Autodesk Inventor part; units mm, degrees
(part 2 of 3)
  arc A282 (85.8723, 45.9613) -> (86.1263, 45.7073) centre (86.1263, 45.9613) ccw
  arc A283 (86.1263, 59.7027) -> (85.8723, 59.4487) centre (86.1263, 59.4487) ccw
  line L431 (85.8723, 45.7073) -> (99.8677, 59.7027) construction
  arc A284 (-19.1948, 59.4487) -> (-19.4488, 59.7027) centre (-19.4488, 59.4487) ccw
  arc A285 (-32.9362, 59.7027) -> (-33.1902, 59.4487) centre (-32.9362, 59.4487) ccw
  line L432 (-19.1948, 59.4487) -> (-19.1948, 45.9613)
  line L433 (-32.9362, 59.7027) -> (-19.4488, 59.7027)
  line L434 (-33.1902, 45.9613) -> (-33.1902, 59.4487)
  line L435 (-19.4488, 45.7073) -> (-32.9362, 45.7073)
  line L436 (-33.1902, 45.7073) -> (-19.1948, 59.7027) construction
  arc A286 (-19.4488, 45.7073) -> (-19.1948, 45.9613) centre (-19.4488, 45.9613) ccw
  arc A287 (-33.1902, 45.9613) -> (-32.9362, 45.7073) centre (-32.9362, 45.9613) ccw
  line L437 (-19.1948, 45.7073) -> (-33.1902, 59.7027) construction
  line L438 (-43.0073, 59.4487) -> (-43.0073, 45.9613)
  arc A288 (-43.2613, 45.7073) -> (-43.0073, 45.9613) centre (-43.2613, 45.9613) ccw
  arc A289 (-43.0073, 59.4487) -> (-43.2613, 59.7027) centre (-43.2613, 59.4487) ccw
  line L439 (-56.7487, 59.7027) -> (-43.2613, 59.7027)
  line L440 (-43.2613, 45.7073) -> (-56.7487, 45.7073)
  line L441 (-57.0027, 45.7073) -> (-43.0073, 59.7027) construction
  line L442 (-43.0073, 45.7073) -> (-57.0027, 59.7027) construction
  arc A290 (-56.7487, 59.7027) -> (-57.0027, 59.4487) centre (-56.7487, 59.4487) ccw
  line L443 (-57.0027, 45.9613) -> (-57.0027, 59.4487)
  arc A291 (-57.0027, 45.9613) -> (-56.7487, 45.7073) centre (-56.7487, 45.9613) ccw
  line L444 (-66.8198, 59.4487) -> (-66.8198, 45.9613)
  arc A292 (-67.0738, 45.7073) -> (-66.8198, 45.9613) centre (-67.0738, 45.9613) ccw
  arc A293 (-66.8198, 59.4487) -> (-67.0738, 59.7027) centre (-67.0738, 59.4487) ccw
  line L445 (-80.5612, 59.7027) -> (-67.0738, 59.7027)
  line L446 (-67.0738, 45.7073) -> (-80.5612, 45.7073)
  line L447 (-80.8152, 45.7073) -> (-66.8198, 59.7027) construction
  line L448 (-66.8198, 45.7073) -> (-80.8152, 59.7027) construction
  arc A294 (-80.5612, 59.7027) -> (-80.8152, 59.4487) centre (-80.5612, 59.4487) ccw
  line L449 (-80.8152, 45.9613) -> (-80.8152, 59.4487)
  arc A295 (-80.8152, 45.9613) -> (-80.5612, 45.7073) centre (-80.5612, 45.9613) ccw
  line L450 (-104.3737, 59.7027) -> (-90.8863, 59.7027)
  arc A296 (-104.3737, 59.7027) -> (-104.6277, 59.4487) centre (-104.3737, 59.4487) ccw
  arc A297 (-90.6323, 59.4487) -> (-90.8863, 59.7027) centre (-90.8863, 59.4487) ccw
  line L451 (-90.6323, 59.4487) -> (-90.6323, 45.9613)
  line L452 (-104.6277, 45.9613) -> (-104.6277, 59.4487)
  line L453 (-104.6277, 45.7073) -> (-90.6323, 59.7027) construction
  line L454 (-90.6323, 45.7073) -> (-104.6277, 59.7027) construction
  arc A298 (-90.8863, 45.7073) -> (-90.6323, 45.9613) centre (-90.8863, 45.9613) ccw
  line L455 (-90.8863, 45.7073) -> (-104.3737, 45.7073)
  arc A299 (-104.6277, 45.9613) -> (-104.3737, 45.7073) centre (-104.3737, 45.9613) ccw
  line L456 (183.1975, 52.705) -> (164.3075, 52.705) construction
  arc A300 (-121.5898, -16.7513) -> (-121.8438, -16.4973) centre (-121.8438, -16.7513) ccw
  line L457 (-121.5898, -16.7513) -> (-121.5898, -30.2387)
  arc A301 (-121.8438, -30.4927) -> (-121.5898, -30.2387) centre (-121.8438, -30.2387) ccw
  line L458 (-135.3312, -16.4973) -> (-121.8438, -16.4973)
  line L459 (-121.8438, -30.4927) -> (-135.3312, -30.4927)
  line L460 (-121.5898, -30.4927) -> (-135.5852, -16.4973) construction
  line L461 (-135.5852, -30.4927) -> (-121.5898, -16.4973) construction
  arc A302 (-135.5852, -30.2387) -> (-135.3312, -30.4927) centre (-135.3312, -30.2387) ccw
  line L462 (-135.5852, -30.2387) -> (-135.5852, -16.7513)
  arc A303 (-135.3312, -16.4973) -> (-135.5852, -16.7513) centre (-135.3312, -16.7513) ccw
  arc A304 (-121.5898, 2.2987) -> (-121.8438, 2.5527) centre (-121.8438, 2.2987) ccw
  arc A305 (-135.3312, 2.5527) -> (-135.5852, 2.2987) centre (-135.3312, 2.2987) ccw
  line L463 (-121.5898, 2.2987) -> (-121.5898, -11.1887)
  line L464 (-121.8438, -11.4427) -> (-135.3312, -11.4427)
  arc A306 (-121.8438, -11.4427) -> (-121.5898, -11.1887) centre (-121.8438, -11.1887) ccw
  line L465 (-121.5898, -11.4427) -> (-135.5852, 2.5527) construction
  line L466 (-135.5852, -11.4427) -> (-121.5898, 2.5527) construction
  line L467 (-135.5852, -11.1887) -> (-135.5852, 2.2987)
  arc A307 (-135.5852, -11.1887) -> (-135.3312, -11.4427) centre (-135.3312, -11.1887) ccw
  line L468 (-135.3312, 2.5527) -> (-121.8438, 2.5527)
  arc A308 (-121.5898, 21.3487) -> (-121.8438, 21.6027) centre (-121.8438, 21.3487) ccw
  arc A309 (-135.3312, 21.6027) -> (-135.5852, 21.3487) centre (-135.3312, 21.3487) ccw
  line L469 (-121.5898, 21.3487) -> (-121.5898, 7.8613)
  line L470 (-121.8438, 7.6073) -> (-135.3312, 7.6073)
  arc A310 (-121.8438, 7.6073) -> (-121.5898, 7.8613) centre (-121.8438, 7.8613) ccw
  line L471 (-121.5898, 7.6073) -> (-135.5852, 21.6027) construction
  line L472 (-135.5852, 7.6073) -> (-121.5898, 21.6027) construction
  line L473 (-135.5852, 7.8613) -> (-135.5852, 21.3487)
  arc A311 (-135.5852, 7.8613) -> (-135.3312, 7.6073) centre (-135.3312, 7.8613) ccw
  line L474 (-135.3312, 21.6027) -> (-121.8438, 21.6027)
  arc A312 (-121.5898, 40.3987) -> (-121.8438, 40.6527) centre (-121.8438, 40.3987) ccw
  arc A313 (-135.3312, 40.6527) -> (-135.5852, 40.3987) centre (-135.3312, 40.3987) ccw
  line L475 (-121.5898, 40.3987) -> (-121.5898, 26.9113)
  line L476 (-121.8438, 26.6573) -> (-135.3312, 26.6573)
  arc A314 (-121.8438, 26.6573) -> (-121.5898, 26.9113) centre (-121.8438, 26.9113) ccw
  line L477 (-121.5898, 26.6573) -> (-135.5852, 40.6527) construction
  line L478 (-135.5852, 26.6573) -> (-121.5898, 40.6527) construction
  line L479 (-135.5852, 26.9113) -> (-135.5852, 40.3987)
  arc A315 (-135.5852, 26.9113) -> (-135.3312, 26.6573) centre (-135.3312, 26.9113) ccw
  line L480 (-135.3312, 40.6527) -> (-121.8438, 40.6527)
  arc A316 (-121.5898, 59.4487) -> (-121.8438, 59.7027) centre (-121.8438, 59.4487) ccw
  arc A317 (-135.3312, 59.7027) -> (-135.5852, 59.4487) centre (-135.3312, 59.4487) ccw
  line L481 (-121.5898, 59.4487) -> (-121.5898, 45.9613)
  line L482 (-121.8438, 45.7073) -> (-135.3312, 45.7073)
  arc A318 (-121.8438, 45.7073) -> (-121.5898, 45.9613) centre (-121.8438, 45.9613) ccw
  line L483 (-121.5898, 45.7073) -> (-135.5852, 59.7027) construction
  line L484 (-135.5852, 45.7073) -> (-121.5898, 59.7027) construction
  line L485 (-135.5852, 45.9613) -> (-135.5852, 59.4487)
  arc A319 (-135.5852, 45.9613) -> (-135.3312, 45.7073) centre (-135.3312, 45.9613) ccw
  line L486 (-135.3312, 59.7027) -> (-121.8438, 59.7027)
  arc A320 (-140.6398, -16.7513) -> (-140.8938, -16.4973) centre (-140.8938, -16.7513) ccw
  arc A321 (-154.3812, -16.4973) -> (-154.6352, -16.7513) centre (-154.3812, -16.7513) ccw
  line L487 (-140.6398, -16.7513) -> (-140.6398, -30.2387)
  line L488 (-140.8938, -30.4927) -> (-154.3812, -30.4927)
  arc A322 (-140.8938, -30.4927) -> (-140.6398, -30.2387) centre (-140.8938, -30.2387) ccw
  line L489 (-140.6398, -30.4927) -> (-154.6352, -16.4973) construction
  line L490 (-154.6352, -30.4927) -> (-140.6398, -16.4973) construction
  line L491 (-154.6352, -30.2387) -> (-154.6352, -16.7513)
  arc A323 (-154.6352, -30.2387) -> (-154.3812, -30.4927) centre (-154.3812, -30.2387) ccw
  line L492 (-154.3812, -16.4973) -> (-140.8938, -16.4973)
  arc A324 (-140.6398, 2.2987) -> (-140.8938, 2.5527) centre (-140.8938, 2.2987) ccw
  arc A325 (-154.3812, 2.5527) -> (-154.6352, 2.2987) centre (-154.3812, 2.2987) ccw
  line L493 (-140.6398, 2.2987) -> (-140.6398, -11.1887)
  line L494 (-140.8938, -11.4427) -> (-154.3812, -11.4427)
  arc A326 (-140.8938, -11.4427) -> (-140.6398, -11.1887) centre (-140.8938, -11.1887) ccw
  line L495 (-140.6398, -11.4427) -> (-154.6352, 2.5527) construction
  line L496 (-154.6352, -11.4427) -> (-140.6398, 2.5527) construction
  line L497 (-154.6352, -11.1887) -> (-154.6352, 2.2987)
  arc A327 (-154.6352, -11.1887) -> (-154.3812, -11.4427) centre (-154.3812, -11.1887) ccw
  line L498 (-154.3812, 2.5527) -> (-140.8938, 2.5527)
  arc A328 (-140.6398, 21.3487) -> (-140.8938, 21.6027) centre (-140.8938, 21.3487) ccw
  arc A329 (-154.3812, 21.6027) -> (-154.6352, 21.3487) centre (-154.3812, 21.3487) ccw
  line L499 (-140.6398, 21.3487) -> (-140.6398, 7.8613)
  line L500 (-140.8938, 7.6073) -> (-154.3812, 7.6073)
  arc A330 (-140.8938, 7.6073) -> (-140.6398, 7.8613) centre (-140.8938, 7.8613) ccw
  line L501 (-140.6398, 7.6073) -> (-154.6352, 21.6027) construction
  line L502 (-154.6352, 7.6073) -> (-140.6398, 21.6027) construction
  line L503 (-154.6352, 7.8613) -> (-154.6352, 21.3487)
  arc A331 (-154.6352, 7.8613) -> (-154.3812, 7.6073) centre (-154.3812, 7.8613) ccw
  line L504 (-154.3812, 21.6027) -> (-140.8938, 21.6027)
  arc A332 (-140.6398, 40.3987) -> (-140.8938, 40.6527) centre (-140.8938, 40.3987) ccw
  arc A333 (-154.3812, 40.6527) -> (-154.6352, 40.3987) centre (-154.3812, 40.3987) ccw
  line L505 (-140.6398, 40.3987) -> (-140.6398, 26.9113)
  line L506 (-140.8938, 26.6573) -> (-154.3812, 26.6573)
  arc A334 (-140.8938, 26.6573) -> (-140.6398, 26.9113) centre (-140.8938, 26.9113) ccw
  line L507 (-140.6398, 26.6573) -> (-154.6352, 40.6527) construction
  line L508 (-154.6352, 26.6573) -> (-140.6398, 40.6527) construction
  line L509 (-154.6352, 26.9113) -> (-154.6352, 40.3987)
  arc A335 (-154.6352, 26.9113) -> (-154.3812, 26.6573) centre (-154.3812, 26.9113) ccw
  line L510 (-154.3812, 40.6527) -> (-140.8938, 40.6527)
  arc A336 (-140.6398, 59.4487) -> (-140.8938, 59.7027) centre (-140.8938, 59.4487) ccw
  arc A337 (-154.3812, 59.7027) -> (-154.6352, 59.4487) centre (-154.3812, 59.4487) ccw
  line L511 (-140.6398, 59.4487) -> (-140.6398, 45.9613)
  line L512 (-140.8938, 45.7073) -> (-154.3812, 45.7073)
  arc A338 (-140.8938, 45.7073) -> (-140.6398, 45.9613) centre (-140.8938, 45.9613) ccw
  line L513 (-140.6398, 45.7073) -> (-154.6352, 59.7027) construction
  line L514 (-154.6352, 45.7073) -> (-140.6398, 59.7027) construction
  line L515 (-154.6352, 45.9613) -> (-154.6352, 59.4487)
  arc A339 (-154.6352, 45.9613) -> (-154.3812, 45.7073) centre (-154.3812, 45.9613) ccw
  line L516 (-154.3812, 59.7027) -> (-140.8938, 59.7027)
  arc A340 (-159.6898, -16.7513) -> (-159.9438, -16.4973) centre (-159.9438, -16.7513) ccw
  arc A341 (-173.4312, -16.4973) -> (-173.6852, -16.7513) centre (-173.4312, -16.7513) ccw
  line L517 (-159.6898, -16.7513) -> (-159.6898, -30.2387)
  line L518 (-159.9438, -30.4927) -> (-173.4312, -30.4927)
  arc A342 (-159.9438, -30.4927) -> (-159.6898, -30.2387) centre (-159.9438, -30.2387) ccw
  line L519 (-159.6898, -30.4927) -> (-173.6852, -16.4973) construction
  line L520 (-173.6852, -30.4927) -> (-159.6898, -16.4973) construction
  line L521 (-173.6852, -30.2387) -> (-173.6852, -16.7513)
  arc A343 (-173.6852, -30.2387) -> (-173.4312, -30.4927) centre (-173.4312, -30.2387) ccw
  line L522 (-173.4312, -16.4973) -> (-159.9438, -16.4973)
  arc A344 (-159.6898, 2.2987) -> (-159.9438, 2.5527) centre (-159.9438, 2.2987) ccw
  arc A345 (-173.4312, 2.5527) -> (-173.6852, 2.2987) centre (-173.4312, 2.2987) ccw
  line L523 (-159.6898, 2.2987) -> (-159.6898, -11.1887)
  line L524 (-159.9438, -11.4427) -> (-173.4312, -11.4427)
  arc A346 (-159.9438, -11.4427) -> (-159.6898, -11.1887) centre (-159.9438, -11.1887) ccw
  line L525 (-159.6898, -11.4427) -> (-173.6852, 2.5527) construction
  line L526 (-173.6852, -11.4427) -> (-159.6898, 2.5527) construction
  line L527 (-173.6852, -11.1887) -> (-173.6852, 2.2987)
  arc A347 (-173.6852, -11.1887) -> (-173.4312, -11.4427) centre (-173.4312, -11.1887) ccw
  line L528 (-173.4312, 2.5527) -> (-159.9438, 2.5527)
  arc A348 (-159.6898, 21.3487) -> (-159.9438, 21.6027) centre (-159.9438, 21.3487) ccw
  arc A349 (-173.4312, 21.6027) -> (-173.6852, 21.3487) centre (-173.4312, 21.3487) ccw
  line L529 (-159.6898, 21.3487) -> (-159.6898, 7.8613)
  line L530 (-159.9438, 7.6073) -> (-173.4312, 7.6073)
  arc A350 (-159.9438, 7.6073) -> (-159.6898, 7.8613) centre (-159.9438, 7.8613) ccw
  line L531 (-159.6898, 7.6073) -> (-173.6852, 21.6027) construction
  line L532 (-173.6852, 7.6073) -> (-159.6898, 21.6027) construction
  line L533 (-173.6852, 7.8613) -> (-173.6852, 21.3487)
  arc A351 (-173.6852, 7.8613) -> (-173.4312, 7.6073) centre (-173.4312, 7.8613) ccw
  line L534 (-173.4312, 21.6027) -> (-159.9438, 21.6027)
  arc A352 (-159.6898, 40.3987) -> (-159.9438, 40.6527) centre (-159.9438, 40.3987) ccw
  arc A353 (-173.4312, 40.6527) -> (-173.6852, 40.3987) centre (-173.4312, 40.3987) ccw
  line L535 (-159.6898, 40.3987) -> (-159.6898, 26.9113)
  line L536 (-159.9438, 26.6573) -> (-173.4312, 26.6573)
  arc A354 (-159.9438, 26.6573) -> (-159.6898, 26.9113) centre (-159.9438, 26.9113) ccw
  line L537 (-159.6898, 26.6573) -> (-173.6852, 40.6527) construction
  line L538 (-173.6852, 26.6573) -> (-159.6898, 40.6527) construction
  line L539 (-173.6852, 26.9113) -> (-173.6852, 40.3987)
  arc A355 (-173.6852, 26.9113) -> (-173.4312, 26.6573) centre (-173.4312, 26.9113) ccw
  line L540 (-173.4312, 40.6527) -> (-159.9438, 40.6527)
  arc A356 (-159.6898, 59.4487) -> (-159.9438, 59.7027) centre (-159.9438, 59.4487) ccw
  arc A357 (-173.4312, 59.7027) -> (-173.6852, 59.4487) centre (-173.4312, 59.4487) ccw
  line L541 (-159.6898, 59.4487) -> (-159.6898, 45.9613)
  line L542 (-159.9438, 45.7073) -> (-173.4312, 45.7073)
  arc A358 (-159.9438, 45.7073) -> (-159.6898, 45.9613) centre (-159.9438, 45.9613) ccw
  line L543 (-159.6898, 45.7073) -> (-173.6852, 59.7027) construction
  line L544 (-173.6852, 45.7073) -> (-159.6898, 59.7027) construction
  line L545 (-173.6852, 45.9613) -> (-173.6852, 59.4487)
  arc A359 (-173.6852, 45.9613) -> (-173.4312, 45.7073) centre (-173.4312, 45.9613) ccw
  line L546 (-173.4312, 59.7027) -> (-159.9438, 59.7027)
  line L547 (-100.0125, -23.495) -> (-183.1975, -23.495) construction
  line L548 (24.5491, 47.3329) -> (18.0571, 47.3329)
  line L549 (17.8031, 47.5869) -> (17.8031, 58.5089)
  line L550 (18.0571, 58.7629) -> (24.5491, 58.7629)
  line L551 (24.8031, 58.5089) -> (24.8031, 47.5869)
  line L552 (21.3031, 47.3329) -> (21.3031, 52.705) construction
  line L553 (33.3375, 59.7027) -> (33.3375, 45.7073) construction
  line L554 (42.1259, 47.3329) -> (48.6179, 47.3329)
  line L555 (48.8719, 47.5869) -> (48.8719, 58.5089)
  line L556 (48.6179, 58.7629) -> (42.1259, 58.7629)
  line L557 (41.8719, 58.5089) -> (41.8719, 47.5869)
  line L558 (45.3719, 47.3329) -> (45.3719, 52.705) construction
  line L559 (150.1648, 26.9113) -> (150.1648, 40.3987)
  line L560 (150.4188, 40.6527) -> (163.9062, 40.6527)
  line L561 (164.1602, 26.6573) -> (150.1648, 40.6527) construction
  line L562 (164.1602, 40.6527) -> (150.1648, 26.6573) construction
  line L563 (148.3741, 28.2829) -> (141.8821, 28.2829)
  line L564 (141.6281, 28.5369) -> (141.6281, 39.4589)
  line L565 (141.8821, 39.7129) -> (148.3741, 39.7129)
  line L566 (148.6281, 39.4589) -> (148.6281, 28.5369)
  line L567 (145.1281, 28.2829) -> (145.1281, 33.655) construction
  line L568 (157.1625, 33.655) -> (145.1281, 33.655) construction
  line L569 (157.1625, 26.6573) -> (157.1625, 40.6527) construction
  line L570 (172.4429, 39.7129) -> (165.9509, 39.7129)
  line L571 (172.6969, 28.5369) -> (172.6969, 39.4589)
  line L572 (169.1969, 28.2829) -> (169.1969, 33.655) construction
  line L573 (165.9509, 28.2829) -> (172.4429, 28.2829)
  line L574 (165.6969, 39.4589) -> (165.6969, 28.5369)
  line L575 (11.1835, 47.3329) -> (4.6915, 47.3329)
  line L576 (4.4375, 47.5869) -> (4.4375, 58.5089)
  line L577 (4.6915, 58.7629) -> (11.1835, 58.7629)
  line L578 (11.4375, 58.5089) -> (11.4375, 47.5869)
  line L579 (7.9375, 47.3329) -> (7.9375, 58.7629) construction
  line L580 (55.4915, 47.3329) -> (61.9835, 47.3329)
  line L581 (62.2375, 47.5869) -> (62.2375, 58.5089)
  line L582 (61.9835, 58.7629) -> (55.4915, 58.7629)
  line L583 (55.2375, 58.5089) -> (55.2375, 47.5869)
  line L584 (58.7375, 47.3329) -> (58.7375, 58.7629) construction
  line L585 (150.4188, 26.6573) -> (163.9062, 26.6573)
  line L586 (164.1602, 40.3987) -> (164.1602, 26.9113)
  arc A360 (163.9062, 26.6573) -> (164.1602, 26.9113) centre (163.9062, 26.9113) ccw
  arc A361 (164.1602, 40.3987) -> (163.9062, 40.6527) centre (163.9062, 40.3987) ccw
  arc A362 (150.4188, 40.6527) -> (150.1648, 40.3987) centre (150.4188, 40.3987) ccw
  arc A363 (150.1648, 26.9113) -> (150.4188, 26.6573) centre (150.4188, 26.9113) ccw
  arc A364 (172.4429, 28.2829) -> (172.6969, 28.5369) centre (172.4429, 28.5369) ccw
  arc A365 (172.6969, 39.4589) -> (172.4429, 39.7129) centre (172.4429, 39.4589) ccw
  arc A366 (165.9509, 39.7129) -> (165.6969, 39.4589) centre (165.9509, 39.4589) ccw
  arc A367 (165.6969, 28.5369) -> (165.9509, 28.2829) centre (165.9509, 28.5369) ccw
  arc A368 (148.3741, 28.2829) -> (148.6281, 28.5369) centre (148.3741, 28.5369) ccw
  arc A369 (148.6281, 39.4589) -> (148.3741, 39.7129) centre (148.3741, 39.4589) ccw
  arc A370 (141.8821, 39.7129) -> (141.6281, 39.4589) centre (141.8821, 39.4589) ccw
  arc A371 (141.6281, 28.5369) -> (141.8821, 28.2829) centre (141.8821, 28.5369) ccw
  line L587 (40.0812, 45.7073) -> (26.5938, 45.7073)
  line L588 (26.3398, 45.9613) -> (26.3398, 59.4487)
  line L589 (26.5938, 59.7027) -> (40.0812, 59.7027)
  line L590 (40.3352, 59.4487) -> (40.3352, 45.9613)
  line L591 (40.3352, 45.7073) -> (26.3398, 59.7027) construction
  line L592 (40.3352, 59.7027) -> (26.3398, 45.7073) construction
  arc A372 (40.0812, 45.7073) -> (40.3352, 45.9613) centre (40.0812, 45.9613) ccw
  arc A373 (40.3352, 59.4487) -> (40.0812, 59.7027) centre (40.0812, 59.4487) ccw
  arc A374 (26.5938, 59.7027) -> (26.3398, 59.4487) centre (26.5938, 59.4487) ccw
  arc A375 (26.3398, 45.9613) -> (26.5938, 45.7073) centre (26.5938, 45.9613) ccw
  arc A376 (48.6179, 47.3329) -> (48.8719, 47.5869) centre (48.6179, 47.5869) ccw
  arc A377 (48.8719, 58.5089) -> (48.6179, 58.7629) centre (48.6179, 58.5089) ccw
  arc A378 (42.1259, 58.7629) -> (41.8719, 58.5089) centre (42.1259, 58.5089) ccw
  arc A379 (41.8719, 47.5869) -> (42.1259, 47.3329) centre (42.1259, 47.5869) ccw
  arc A380 (24.5491, 47.3329) -> (24.8031, 47.5869) centre (24.5491, 47.5869) ccw
  arc A381 (17.8031, 47.5869) -> (18.0571, 47.3329) centre (18.0571, 47.5869) ccw
  arc A382 (18.0571, 58.7629) -> (17.8031, 58.5089) centre (18.0571, 58.5089) ccw
  arc A383 (24.8031, 58.5089) -> (24.5491, 58.7629) centre (24.5491, 58.5089) ccw
  arc A384 (11.1835, 47.3329) -> (11.4375, 47.5869) centre (11.1835, 47.5869) ccw
  arc A385 (4.4375, 47.5869) -> (4.6915, 47.3329) centre (4.6915, 47.5869) ccw
  arc A386 (4.6915, 58.7629) -> (4.4375, 58.5089) centre (4.6915, 58.5089) ccw
  arc A387 (11.4375, 58.5089) -> (11.1835, 58.7629) centre (11.1835, 58.5089) ccw
  arc A388 (55.2375, 47.5869) -> (55.4915, 47.3329) centre (55.4915, 47.5869) ccw
  arc A389 (61.9835, 47.3329) -> (62.2375, 47.5869) centre (61.9835, 47.5869) ccw
  arc A390 (62.2375, 58.5089) -> (61.9835, 58.7629) centre (61.9835, 58.5089) ccw
  arc A391 (55.4915, 58.7629) -> (55.2375, 58.5089) centre (55.4915, 58.5089) ccw
  line L593 (21.3031, 52.705) -> (33.3375, 52.705) construction
  line L594 (-83.7438, 26.6573) -> (-97.2312, 26.6573)
  line L595 (-97.4852, 26.9113) -> (-97.4852, 40.3987)
  line L596 (-97.2312, 40.6527) -> (-83.7438, 40.6527)
  line L597 (-83.4898, 40.3987) -> (-83.4898, 26.9113)
  line L598 (-83.4898, 26.6573) -> (-97.4852, 40.6527) construction
  line L599 (-97.4852, 26.6573) -> (-83.4898, 40.6527) construction
  arc A392 (-83.7438, 26.6573) -> (-83.4898, 26.9113) centre (-83.7438, 26.9113) ccw
  arc A393 (-97.4852, 26.9113) -> (-97.2312, 26.6573) centre (-97.2312, 26.9113) ccw
  arc A394 (-97.2312, 40.6527) -> (-97.4852, 40.3987) centre (-97.2312, 40.3987) ccw
  arc A395 (-83.4898, 40.3987) -> (-83.7438, 40.6527) centre (-83.7438, 40.3987) ccw
  line L600 (-90.4875, 26.6573) -> (-90.4875, 40.6527) construction
  line L601 (-99.2759, 28.2829) -> (-105.7679, 28.2829)
  line L602 (-106.0219, 28.5369) -> (-106.0219, 39.4589)
  line L603 (-105.7679, 39.7129) -> (-99.2759, 39.7129)
  line L604 (-99.0219, 39.4589) -> (-99.0219, 28.5369)
  arc A396 (-99.2759, 28.2829) -> (-99.0219, 28.5369) centre (-99.2759, 28.5369) ccw
  arc A397 (-106.0219, 28.5369) -> (-105.7679, 28.2829) centre (-105.7679, 28.5369) ccw
  arc A398 (-105.7679, 39.7129) -> (-106.0219, 39.4589) centre (-105.7679, 39.4589) ccw
  arc A399 (-99.0219, 39.4589) -> (-99.2759, 39.7129) centre (-99.2759, 39.4589) ccw
  line L605 (-81.6991, 28.2829) -> (-75.2071, 28.2829)
  line L606 (-74.9531, 28.5369) -> (-74.9531, 39.4589)
  line L607 (-75.2071, 39.7129) -> (-81.6991, 39.7129)
  line L608 (-81.9531, 39.4589) -> (-81.9531, 28.5369)
  arc A400 (-81.9531, 28.5369) -> (-81.6991, 28.2829) centre (-81.6991, 28.5369) ccw
  arc A401 (-75.2071, 28.2829) -> (-74.9531, 28.5369) centre (-75.2071, 28.5369) ccw
  arc A402 (-74.9531, 39.4589) -> (-75.2071, 39.7129) centre (-75.2071, 39.4589) ccw
  arc A403 (-81.6991, 39.7129) -> (-81.9531, 39.4589) centre (-81.6991, 39.4589) ccw
  line L609 (-78.4531, 28.2829) -> (-78.4531, 33.655) construction
  line L610 (-102.5219, 28.2829) -> (-102.5219, 33.655) construction
  line L611 (-102.5219, 33.655) -> (-78.4531, 33.655) construction
  arc A404 (-90.6323, 11.8237) -> (-90.8863, 12.0777) centre (-90.8863, 11.8237) ccw
  line L612 (-90.6323, 11.8237) -> (-90.6323, -1.6637)
  arc A405 (-90.8863, -1.9177) -> (-90.6323, -1.6637) centre (-90.8863, -1.6637) ccw
  line L613 (-104.3737, 12.0777) -> (-90.8863, 12.0777)
  line L614 (-90.8863, -1.9177) -> (-104.3737, -1.9177)
  line L615 (-90.6323, -1.9177) -> (-104.6277, 12.0777) construction
  line L616 (-104.6277, -1.9177) -> (-90.6323, 12.0777) construction
  arc A406 (-104.6277, -1.6637) -> (-104.3737, -1.9177) centre (-104.3737, -1.6637) ccw
  line L617 (-104.6277, -1.6637) -> (-104.6277, 11.8237)
  arc A407 (-104.3737, 12.0777) -> (-104.6277, 11.8237) centre (-104.3737, 11.8237) ccw
  line L618 (-92.5119, -10.2616) -> (-103.4339, -10.2616)
  line L619 (-103.6879, -10.0076) -> (-103.6879, -3.7084)
  line L620 (-103.4339, -3.4544) -> (-92.5119, -3.4544)
  line L621 (-92.2579, -3.7084) -> (-92.2579, -10.0076)
  line L622 (-92.2579, -6.858) -> (-97.63, -6.858) construction
  line L623 (-90.6323, 5.08) -> (-104.6277, 5.08) construction
  line L624 (-97.63, -6.858) -> (-97.63, 5.08) construction
  arc A408 (-92.5119, -10.2616) -> (-92.2579, -10.0076) centre (-92.5119, -10.0076) ccw
  arc A409 (-103.6879, -10.0076) -> (-103.4339, -10.2616) centre (-103.4339, -10.0076) ccw
  arc A410 (-103.4339, -3.4544) -> (-103.6879, -3.7084) centre (-103.4339, -3.7084) ccw
  arc A411 (-92.2579, -3.7084) -> (-92.5119, -3.4544) centre (-92.5119, -3.7084) ccw
  line L625 (-92.5119, 20.4216) -> (-103.4339, 20.4216)
  line L626 (-103.6879, 20.1676) -> (-103.6879, 13.8684)
  line L627 (-103.4339, 13.6144) -> (-92.5119, 13.6144)
  line L628 (-92.2579, 13.8684) -> (-92.2579, 20.1676)
  line L629 (-92.2579, 17.018) -> (-97.63, 17.018) construction
  arc A412 (-92.2579, 20.1676) -> (-92.5119, 20.4216) centre (-92.5119, 20.1676) ccw
  arc A413 (-103.4339, 20.4216) -> (-103.6879, 20.1676) centre (-103.4339, 20.1676) ccw
  arc A414 (-103.6879, 13.8684) -> (-103.4339, 13.6144) centre (-103.4339, 13.8684) ccw
  arc A415 (-92.5119, 13.6144) -> (-92.2579, 13.8684) centre (-92.5119, 13.8684) ccw
  point P0 (0, 0)
  point P1 (0, 0)
  point P2 (166.6875, -23.495)
  point P3 (69.9269, -109.0243)
  point P4 (166.6875, -52.07)
  point P5 (166.6875, -52.07)
  point P6 (147.6375, -23.495)
  point P7 (128.5875, -23.495)
  point P8 (109.5375, -23.495)
  point P9 (90.4875, -23.495)
  point P10 (71.4375, -23.495)
  point P11 (52.3875, -23.495)
  point P12 (33.3375, -23.495)
  point P13 (14.2875, -23.495)
  point P14 (-4.7625, -23.495)
  point P15 (-23.8125, -23.495)
  point P16 (-42.8625, -23.495)
  point P17 (-61.9125, -23.495)
  point P18 (-80.9625, -23.495)
  point P19 (166.6875, -23.495)
  point P20 (138.1125, -4.445)
  point P21 (119.0625, -4.445)
  point P22 (100.0125, -4.445)
  point P23 (80.9625, -4.445)
  point P24 (61.9125, -4.445)
  point P25 (42.8625, -4.445)
  point P26 (23.8125, -4.445)
  point P27 (4.7625, -4.445)
  point P28 (-14.2875, -4.445)
  point P29 (-33.3375, -4.445)
  point P30 (-52.3875, -4.445)
  point P31 (-71.4375, -4.445)
  point P32 (133.35, 14.605)
  point P33 (114.3, 14.605)
  point P34 (95.25, 14.605)
  point P35 (76.2, 14.605)
  point P36 (57.15, 14.605)
  point P37 (38.1, 14.605)
  point P38 (19.05, 14.605)
  point P39 (0, 14.605)
  point P40 (-19.05, 14.605)
  point P41 (-38.1, 14.605)
  point P42 (-57.15, 14.605)
  point P43 (-76.2, 14.605)
  point P44 (159.5425, 14.605)
  point P45 (159.5425, 14.605)
  point P46 (161.925, -4.445)
  point P47 (161.925, -4.445)
  point P48 (109.5375, 33.655)
  point P49 (90.4875, 33.655)
  point P50 (71.4375, 33.655)
  point P51 (52.3875, 33.655)
  point P52 (33.3375, 33.655)
  point P53 (14.2875, 33.655)
  point P54 (-4.7625, 33.655)
  point P55 (-23.8125, 33.655)
  point P56 (-42.8625, 33.655)
  point P57 (-61.9125, 33.655)
  point P58 (140.495, 52.705)
  point P59 (116.6825, 52.705)
  point P60 (92.87, 52.705)
  point P61 (-26.1925, 52.705)
  point P62 (-50.005, 52.705)
  point P63 (-73.8175, 52.705)
  point P64 (-97.63, 52.705)
  point P65 (-128.5875, -23.495)
  point P66 (-128.5875, -4.445)
  point P67 (-128.5875, 14.605)
  point P68 (-128.5875, 33.655)
  point P69 (-128.5875, 52.705)
  point P70 (-147.6375, -23.495)
  point P71 (-147.6375, -4.445)
  point P72 (-147.6375, 14.605)
  point P73 (-147.6375, 33.655)
  point P74 (-147.6375, 52.705)
  point P75 (-166.6875, -23.495)
  point P76 (-166.6875, -4.445)
  point P77 (-166.6875, 14.605)
  point P78 (-166.6875, 33.655)
  point P79 (-166.6875, 52.705)
  point P80 (-128.5875, -23.495)
  point P81 (24.8031, 47.3329)
  point P82 (17.8031, 58.7629)
  point P83 (17.8031, 47.3329)
  point P84 (24.8031, 58.7629)
  point P85 (41.8719, 47.3329)
  point P86 (48.8719, 58.7629)
  point P87 (48.8719, 47.3329)
  point P88 (41.8719, 58.7629)
  point P89 (148.6281, 28.2829)
  point P90 (141.6281, 39.7129)
  point P91 (141.6281, 28.2829)
  point P92 (148.6281, 39.7129)
  point P93 (172.6969, 39.7129)
  point P94 (165.6969, 39.7129)
  point P95 (172.6969, 28.2829)
  point P96 (165.6969, 28.2829)
  point P97 (157.1625, 33.655)
  point P98 (-97.63, 5.08)
  point P99 (11.4375, 47.3329)
  point P100 (4.4375, 58.7629)
  point P101 (4.4375, 47.3329)
  point P102 (11.4375, 58.7629)
  point P103 (55.2375, 47.3329)
  point P104 (62.2375, 58.7629)
  point P105 (62.2375, 47.3329)
  point P106 (55.2375, 58.7629)
  point P107 (-90.4875, 33.655)
  point P108 (26.3398, 59.7027)
  point P109 (-83.4898, 40.6527)
  point P110 (-90.4875, 33.655)
  point P111 (-106.0219, 39.7129)
  point P112 (-106.0219, 28.2829)
  point P113 (-99.0219, 39.7129)
  point P114 (-74.9531, 39.7129)
  point P115 (-74.9531, 28.2829)
  point P116 (-81.9531, 39.7129)
  point P117 (-90.4875, 33.655)
  point P118 (-90.4875, 33.655)
  point P119 (-97.63, 5.08)
  point P120 (-103.6879, -3.4544)
  point P121 (-103.6879, -10.2616)
  point P122 (-92.2579, -3.4544)
  point P123 (-103.6879, 13.6144)
  point P124 (-103.6879, 20.4216)
  point P125 (-92.2579, 13.6144)
  point P126 (-97.63, 5.08)
  dimension "d0" = 366.395
  dimension "d1" = 137.16
  dimension "d2" = 3
  dimension "d3" = 13.9954
  dimension "d4" = 13.9954
  dimension "d5" = 0.254
  dimension "d8" = 19.05
  dimension "d15" = 85.725
  dimension "d20" = 54.61
  dimension "d21" = 16.51
  dimension "d26" = 13.9954
  dimension "d27" = 13.9954
  dimension "d28" = 0.254
  dimension "d29" = 13.9954
  dimension "d30" = 13.9954
  dimension "d31" = 0.254
  dimension "d32" = 13.9954
  dimension "d33" = 13.9954
  dimension "d34" = 0.254
  dimension "d35" = 13.9954
  dimension "d36" = 13.9954
  dimension "d37" = 0.254
  dimension "d39" = 28.575
  dimension "d42" = 19.05
  dimension "d47" = 16.51
  dimension "d48" = 13.9954
  dimension "d49" = 13.9954
  dimension "d50" = 0.254
  dimension "d53" = 19.05
  dimension "d58" = 45.085
  dimension "d59" = 19.05
  dimension "d60" = 13.9954
  dimension "d61" = 13.9954
  dimension "d62" = 0.254
  dimension "d65" = 19.05
  dimension "d70" = 49.8475
  dimension "d71" = 23.655
  dimension "d72" = 19.05
  dimension "d73" = 13.9954
  dimension "d74" = 13.9954
  dimension "d75" = 0.254
  dimension "d76" = 21.2725
  dimension "d77" = 13.9954
  dimension "d78" = 13.9954
  dimension "d79" = 0.254
  dimension "d82" = 19.05
  dimension "d87" = 54.61
  dimension "d92" = 19.05
  dimension "d93" = 26.035
  dimension "d94" = 13.9954
  dimension "d95" = 13.9954
  dimension "d96" = 0.254
  dimension "d99" = 23.8125
  dimension "d106" = 190.5
  dimension "d111" = 18.89
  dimension "d112" = 19.05
  dimension "d113" = 13.9954
  dimension "d114" = 13.9954
  dimension "d115" = 0.254
  dimension "d118" = 19.05
  dimension "d121" = 19.05
  dimension "d124" = 28.575
  dimension "d145" = 7
  dimension "d146" = 11.43
  constraints: 1258 end point, 835 point on line, 832 point on circle, 416 centre point, 190 tangent, 74 equal radius, 52 symmetric about line, 47 midpoint, 40 parallel, 39 horizontal, 24 perpendicular, 16 collinear, 7 coincident, 7 vertical, 2105 other
  measures "d0" distance of L5.end L4.start
  measures "d1" distance of L4.end L5.end
  measures "d2" radius of A0
  measures "d3" distance of L10.end L11.end
  measures "d4" distance of L11.start L10.end
  measures "d5" radius of A4
  measures "d8" distance of L10.start L15.start
  measures "d15" distance of L10.end L33.end
  measures "d21" distance between parallel lines of L0 L79
  measures "d26" distance of L84.end L85.end
  measures "d27" distance of L85.start L84.end
  measures "d28" radius of A52
  measures "d29" distance of L90.end L91.end
  measures "d30" distance of L91.start L90.end
  measures "d31" radius of A56
  measures "d32" distance of L96.end L97.end
  measures "d33" distance of L97.start L96.end
  measures "d34" radius of A60
  measures "d35" distance of L101.end L102.end
  measures "d36" distance of L102.start L101.end
  measures "d37" radius of A65
  measures "d39" distance of point (166.688, -52.07) point (166.688, -23.495)
  measures "d42" distance of L84.start L108.start
  measures "d48" distance of L192.end L193.end
  measures "d49" distance of L193.start L192.end
  measures "d50" radius of A127
  measures "d53" distance of L192.end L199.end
  measures "d58" distance of L261.end L261.start
  measures "d59" distance from line of L261 point (166.688, -23.495)
  measures "d60" distance of L265.end L266.end
  measures "d61" distance of L266.start L265.end
  measures "d62" radius of A175
  measures "d65" distance of A174.centre A176.centre
  measures "d70" distance of L334.end L334.start
  measures "d72" distance between parallel lines of L334 L261
  measures "d73" distance of L338.end L339.end
  measures "d74" distance of L339.start L338.end
  measures "d75" radius of A223
  measures "d77" distance of L344.end L345.end
  measures "d78" distance of L345.start L344.end
  measures "d79" radius of A227
  measures "d82" distance of L99.end L349.end
  measures "d87" distance of L407.end L407.start
  measures "d92" distance between parallel lines of L334 L407
  measures "d94" distance of L411.end L412.end
  measures "d95" distance of L412.start L411.end
  measures "d96" radius of A269
  measures "d99" distance of L408.start L414.start
  measures "d106" distance of L408.end L432.end
  measures "d111" distance of L456.end L456.start
  measures "d112" distance between parallel lines of L407 L456
  measures "d113" distance of L460.end L461.end
  measures "d114" distance of L461.start L460.end
  measures "d115" radius of A301
  measures "d118" distance of L458.end L468.end
  measures "d121" distance of L458.end L492.end
  measures "d124" distance of point (-128.587, -23.495) L547.start
  measures "d145" distance of point (17.803, 58.763) point (24.803, 58.763)
  measures "d146" distance of point (17.803, 47.333) point (17.803, 58.763)
extrude "押し出し1" add sketch "スケッチ1" along normal blind 1.524 contours L0 A3 L1 A2 L2 A1 L3 A0 | L469 A310 L470 A311 L473 A309 L474 A308 | L475 A314 L476 A315 L479 A313 L480 A312 | L499 A330 L500 A331 L503 A329 L504 A328 | L529 A350 L530 A351 L533 A349 L534 A348 | L535 A354 L536 A355 L539 A353 L540 A352
fillet "フィレット1" radius 0.1 16 edges at (182.3188, 1.524, 67.7013) (183.1975, 1.524, 0) (182.3188, 1.524, -67.7013) (0, 1.524, -68.58) (-182.3188, 1.524, -67.7013) (-183.1975, 1.524, 0) (-182.3188, 1.524, 67.7013) (0, 1.524, 68.58) (183.1975, 0, 0) (182.3188, 0, -67.7013) (0, 0, -68.58) (-182.3188, 0, -67.7013) (-183.1975, 0, 0) (-182.3188, 0, 67.7013) (0, 0, 68.58) (182.3188, 0, 67.7013)